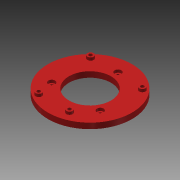
# Autodesk Inventor part: Arduino Mount
Saved by Autodesk Inventor 2014 (Build 180170000, 170)
## iProperties
Created: 2014-02-05
Part Number: Arduino Mount
Material: Generic
Document SubType Name: Modeling
Designer: Spooner
Density: 1 g/cm^3
Appearance: Light Red
Author: Spooner
Autodesk Inventor part; units mm, degrees
ref_plane "YZ Plane" through (0, 0, 0) normal (1, 0, 0) x (0, 1, 0)
ref_plane "XZ Plane" through (0, 0, 0) normal (0, 1, 0) x (-1, 0, 0)
ref_plane "XY Plane" through (0, 0, 0) normal (0, 0, 1) x (1, 0, 0)
sketch "Sketch1" plane through (0, 0, 0) normal (0, 1, 0) x (-1, 0, 0)
  circle A0 centre (0, 0) radius 38.1
  circle A1 centre (0, 0) radius 19.05
  circle A2 centre (0, 0) radius 25.4 construction
  dimension "d0" = 50.8
  dimension "d1" = 6.35
  dimension "d5" = 76.2
  constraints: 3 centre point, 3 coincident
  measures "d0" diameter of A2
  measures "d1" radial gap between concentric circles of A1 A2
  measures "d5" diameter of A0
extrude "Extrusion1" add sketch "Sketch1" along normal blind 5.08
sketch "Sketch2" plane through (0, 5.08, 0) normal (0, 1, 0) x (1, 0, 0)
  circle A0 centre (0, 0) radius 19.05 projected
  point P0 (0, 25.4)
  dimension "d6" = 25.4
  constraints: 1 vertical alignment
  measures "d6" distance of A0.centre point (0, 25.4)
hole "Hole1" at (0, 5.08, -25.4) direction (0, -1, 0) diameter 3.048 end through all counterbore diameter 6.096 counterbore depth 2.54
pattern_circular "Circular Pattern1" count 3 over 360 about axis through (0, 0, 0) along (0, 1, 0) of "Hole1"
sketch "Sketch4" plane through (0, 5.08, 0) normal (0, 1, 0) x (1, 0, 0)
  circle A0 centre (0, 0) radius 19.05 projected
  circle A1 centre (24.7446, 22.7186) radius 1.524
  circle A2 centre (-23.5154, 23.9886) radius 1.524
  circle A3 centre (-18.4354, -28.0814) radius 1.524
  circle A4 centre (9.5046, -28.0814) radius 1.524
  dimension "d17" = 3.048
  dimension "d18" = 27.94
  dimension "d19" = 15.24
  dimension "d20" = 5.08
  dimension "d21" = 50.8
  dimension "d22" = 1.27
  dimension "d23" = 33.5921
  dimension "d24" = 33.5921
  dimension "d25" = 33.5921
  constraints: 4 centre point, 3 equal radius, 1 horizontal alignment
  measures "d17" diameter of A4
  measures "d18" distance of A3.centre A4.centre
  measures "d19" horizontal distance of A4.centre A1.centre
  measures "d20" horizontal distance of A2.centre A3.centre
  measures "d21" vertical distance of A4.centre A1.centre
  measures "d22" vertical distance of A1.centre A2.centre
  measures "d23" distance of A0.centre A2.centre
  measures "d24" distance of A3.centre A0.centre
  measures "d25" distance of A1.centre A0.centre
extrude "Extrusion2" cut sketch "Sketch4" against normal through all contours A1 | A2 | A3 | A4
sketch "Sketch5" plane through (0, 5.08, 0) normal (0, 1, 0) x (1, 0, 0)
  circle A0 centre (-18.4354, -28.0814) radius 1.524 projected
  circle A1 centre (24.7446, 22.7186) radius 1.524 projected
  circle A2 centre (-23.5154, 23.9886) radius 1.524 projected
  circle A3 centre (9.5046, -28.0814) radius 1.524 projected
  circle A4 centre (-23.5154, 23.9886) radius 2.8575
  circle A5 centre (24.7446, 22.7186) radius 2.8575
  circle A6 centre (9.5046, -28.0814) radius 2.8575
  circle A7 centre (-18.4354, -28.0814) radius 2.8575
  dimension "d28" = 5.715
  constraints: 4 centre point, 4 coincident, 3 equal radius
  measures "d28" diameter of A7
extrude "Extrusion3" add sketch "Sketch5" along normal blind 2.54
equation "\"d23\" = d25"
equation "\"d24\" = d25"
body "Solid1"
